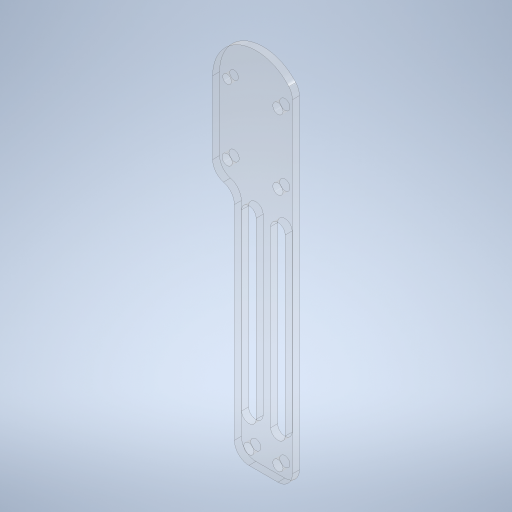
# Autodesk Inventor part: Side Plate
Saved by Autodesk Inventor 2024 (Build 280153000, 153)
## iProperties
Created: 2023-12-18
Part Number: Side Plate
Material: Generic
Document SubType Name: Sheet Metal
Designer: greg
Density: 1 g/cm^3
Sheet Metal Rule: Default
Appearance: Polycarbonate - Clear
Author: greg
Autodesk Inventor part; units mm, degrees
ref_plane "YZ Plane" through (0, 0, 0) normal (1, 0, 0) x (0, 1, 0)
ref_plane "XZ Plane" through (0, 0, 0) normal (0, 1, 0) x (-1, 0, 0)
ref_plane "XY Plane" through (0, 0, 0) normal (0, 0, 1) x (1, 0, 0)
sketch "Sketch1" plane through (0, 0, 0) normal (0, 0, 1) x (1, 0, 0)
  line L0 (0, 0) -> (25.4, 0)
  line L1 (25.4, 0) -> (25.4, 101.6)
  line L2 (25.4, 101.6) -> (0, 101.6)
  line L3 (0, 101.6) -> (0, 0)
  line L4 (6.35, 95.25) -> (6.35, 19.05) construction
  line L5 (3.175, 95.25) -> (3.175, 19.05)
  line L6 (9.525, 19.05) -> (9.525, 95.25)
  arc A0 (9.525, 95.25) -> (3.175, 95.25) centre (6.35, 95.25) ccw
  arc A1 (3.175, 19.05) -> (9.525, 19.05) centre (6.35, 19.05) ccw
  line L7 (19.05, 95.25) -> (19.05, 19.05) construction
  line L8 (15.875, 95.25) -> (15.875, 19.05)
  line L9 (22.225, 19.05) -> (22.225, 95.25)
  arc A2 (22.225, 95.25) -> (15.875, 95.25) centre (19.05, 95.25) ccw
  arc A3 (15.875, 19.05) -> (22.225, 19.05) centre (19.05, 19.05) ccw
  line L10 (6.35, 57.15) -> (19.05, 57.15) construction
  point P0 (12.7, 57.15)
  point P1 (12.7, 0)
  dimension "d2" = 6.35
  dimension "d3" = 76.2
  dimension "d4" = 19.05
  dimension "d5" = 6.35
  dimension "d7" = 12.7
  dimension "d8" = 3.175
  measures "d2" distance between parallel lines of L6 L5
  measures "d3" distance of L4.start L4.end
  measures "d4" distance from line of L0 L4.end
  measures "d5" distance from line of L2 L4.start
  measures "d7" distance of L10.start L10.end
  measures "d8" distance between parallel lines of L1 L9
extrude "Plate1" add sketch "Sketch1" along normal blind 3.048
sketch "Sketch2" plane through (0, 0, 3.048) normal (0, 0, 1) x (1, 0, 0)
  arc A0 (25.4, 150.2303) -> (-9.525, 139.7) centre (9.525, 139.7) ccw
  line L0 (25.4, 0) -> (25.4, 101.6)
  line L1 (25.4, 101.6) -> (0, 101.6)
  line L2 (0, 101.6) -> (-9.525, 101.6)
  line L3 (-9.525, 101.6) -> (-9.525, 139.7)
  line L4 (25.4, 101.6) -> (25.4, 150.2303)
  point P0 (0, 0)
  point P1 (28.575, 139.7)
  dimension "d10" = 38.1
  dimension "d11" = 3.175
  dimension "d12" = 38.1
  dimension "d13" = 34.925
  measures "d10" diameter of A0
  measures "d11" distance from line of L4 point (28.575, 139.7)
  measures "d12" distance from line of L1 A0.centre
  measures "d13" distance between parallel lines of L3 L4
sheet face with bend "Face2" sketch "Sketch2" thickness 3.048 toward (0, 0, -1) bend radius 3.048 relief straight relief width 3.048 relief depth 1.524
bend "Bend1"
fillet "Corner Round1" radius 6.35 5 edges at (-9.525, 101.6, 1.524) (0, 101.6, 1.524) (25.4, 150.2303, 1.524) (0, 0, 1.524) (25.4, 0, 1.524)
sketch "Sketch3" plane through (0, 0, 3.048) normal (0, 0, 1) x (1, 0, 0)
  line L0 (6.35, 6.35) -> (19.05, 6.35) construction
  line L1 (19.05, 0) -> (6.35, 0) projected
  line L2 (25.4, 148.1003) -> (25.4, 6.35) projected
  line L3 (-9.525, 139.7) -> (-9.525, 107.95) projected
  line L4 (-3.175, 111.125) -> (19.05, 111.125) construction
  line L5 (-9.525, 123.825) -> (25.4, 123.825) construction
  point P0 (0, 0)
  point P1 (12.7, 6.35)
  point P2 (12.7, 0)
  point P3 (19.05, 141.605)
  point P4 (-3.175, 141.605)
  point P5 (7.9375, 123.825)
  point P6 (7.9375, 111.125)
  dimension "d20" = 6.35
  dimension "d21" = 6.35
  dimension "d22" = 6.35
  dimension "d23" = 3.175
  dimension "d25" = 30.48
  constraints: 6 end point, 5 midpoint, 4 vertical alignment, 2 horizontal, 1 coincident, 1 horizontal alignment, 1 perpendicular, 1 point on line
  measures "d20" distance between parallel lines of L1 L0
  measures "d21" distance from line of L2 L0.end
  measures "d22" distance from line of L3 L4.start
  measures "d23" distance from line of L3.end L4
  measures "d25" distance of L4.start point (-3.175, 141.605)
hole "Hole1" at (6.35, 6.35, 3.048) at (19.05, 6.35, 3.048) at (-3.175, 111.125, 3.048) at (19.05, 111.125, 3.048) at (19.05, 141.605, 3.048) at (-3.175, 141.605, 3.048) direction (0, 0, -1) diameter 3.81 end through all clearance for "Flat Head Machine Screw (82)" size "#6" standard "Ansi Unified Screw Threads"
sketch "Sketch4" plane through (0, 0, 3.048) normal (0, 0, 1) x (1, 0, 0)
  point P0 (6.35, 6.35)
  point P1 (19.05, 6.35)
  point P2 (19.05, 111.125)
  point P3 (-3.175, 111.125)
  point P4 (19.05, 141.605)
hole "Hole2" at (6.35, 6.35, 3.048) at (19.05, 6.35, 3.048) at (19.05, 111.125, 3.048) at (-3.175, 111.125, 3.048) at (19.05, 141.605, 3.048) direction (0, 0, -1) diameter 4.4958 end through all
equation "\"d31\" = Thickness"
equation "\"d9\" = Thickness"
equation "\"d14\" = BendRadius"
equation "\"d15\" = BendReliefWidth"
equation "\"d17\" = MinimumRemnant"
equation "\"d16\" = BendReliefDepth"
equation "\"d18\" = TransitionRadius"
equation "\"BendRadius\" = Thickness"
equation "\"BendReliefWidth\" = Thickness"
equation "\"BendReliefDepth\" = 0.5 * Thickness"
equation "\"CornerReliefSize\" = 4 * Thickness"
equation "\"MinimumRemnant\" = 2 * Thickness"
equation "\"TransitionRadius\" = BendRadius"
equation "\"JacobiRadiusSize\" = BendRadius"
equation "\"GapSize\" = Thickness"
equation "\"Thickness\" = 3.048"
body "Solid1"
